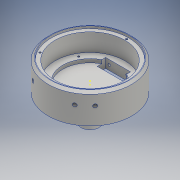
# Autodesk Inventor part: joint_read_side
Saved by Autodesk Inventor 2017 (Build 210142000, 142)
## iProperties
Created: 2017-09-26
Part Number: joint_read_side
Material: Aluminum 6061
Document SubType Name: Modeling
Designer: Thoma
Density: 2.7 g/cm^3
Appearance: Aluminum - Flat
Author: Thoma
Autodesk Inventor part; units mm, degrees
sketch "Sketch1" plane through (0, 0, 0) normal (0, 0, 1) x (1, 0, 0)
  circle A0 centre (0, 0) radius 35
  dimension "d0" = 70
  constraints: 1 centre point, 1 coincident
  measures "d0" diameter of A0
extrude "Extrusion1" add sketch "Sketch1" along normal blind 25
sketch "Sketch2" plane through (0, 0, 25) normal (0, 0, 1) x (1, 0, 0)
  circle A0 centre (0, 0) radius 23.5 construction
  line L0 (0, 0) -> (0, 47.2726) construction
  circle A1 centre (0, 0) radius 29.25
  point P0 (0, 23.5)
  dimension "d3" = 47
  dimension "d173" = 58.5
  constraints: 2 end point, 1 centre point, 1 coincident, 1 vertical, 1 vertical alignment, 2 other
  measures "d173" diameter of A1
extrude "Extrusion2" cut sketch "Sketch2" against normal blind 17
sketch "Sketch4" plane through (0, 0, 8) normal (0, 0, 1) x (1, 0, 0)
  circle A0 centre (0, 0) radius 22.8812
  point P0 (-4.25, 23.5)
  point P1 (4.25, 23.5)
  dimension "d148" = 45.7624
  constraints: 1 centre point
  measures "d148" diameter of A0
extrude "Extrusion4" cut sketch "Sketch4" against normal blind 3
ref_plane "Work Plane1" through (0, 35, 0) normal (0, 1, 0) x (-1, 0, 0)
sketch "Sketch8" plane through (0, 0, 25) normal (0, 0, 1) x (1, 0, 0)
  circle A0 centre (0, 0) radius 32.5
  dimension "d36" = 65
  constraints: 1 centre point, 1 coincident
  measures "d36" diameter of A0
extrude "Extrusion7" cut sketch "Sketch8" against normal blind 2
chamfer "Chamfer1" distance 2 angle 45 1 edges at (-35, 0, 25)
sketch "Sketch10" plane through (0, 0, 8) normal (0, 0, 1) x (1, 0, 0)
  circle A0 centre (0, 0) radius 25.881 construction
  circle A1 centre (0, 0) radius 22.8812 projected
  point P0 (0, -25.881)
  point P1 (-22.4136, 12.9405)
  point P2 (22.4136, 12.9405)
  dimension "d49" = 51.762
  dimension "d52" = 360
  constraints: 2 coincident, 1 vertical alignment, 7 other
hole "Hole3" at (0, -25.881, 8) at (-22.4136, 12.9405, 8) at (22.4136, 12.9405, 8) direction (0, 0, -1) diameter 1.6 depth 5 tip angle 118
sketch "Sketch11" plane through (0, 0, 23) normal (0, 0, 1) x (1, 0, 0)
  circle A0 centre (0, 0) radius 30.6575 construction
  point P0 (0, 30.6575)
  point P1 (-26.5502, -15.3287)
  point P2 (26.5502, -15.3288)
  dimension "d61" = 61.315
  dimension "d64" = 360
  constraints: 1 coincident, 1 vertical alignment, 6 other
hole "Hole4" at (0, 30.6575, 23) at (-26.5502, -15.3287, 23) at (26.5502, -15.3288, 23) direction (0, 0, -1) diameter 1.6 depth 5 tip angle 118
thread "Thread1" size "M1.6x0.35" class "6H" standard "ANSI Metric M Profile" full length
thread "Thread2" size "M1.6x0.35" class "6H" standard "ANSI Metric M Profile" full length
thread "Thread3" size "M1.6x0.35" class "6H" standard "ANSI Metric M Profile" full length
thread "Thread4" size "M1.6x0.35" class "6H" standard "ANSI Metric M Profile" full length
thread "Thread5" size "M1.6x0.35" class "6H" standard "ANSI Metric M Profile" full length
thread "Thread6" size "M1.6x0.35" class "6H" standard "ANSI Metric M Profile" full length
sketch "Sketch12" plane through (0, 0, 0) normal (0, 0, -1) x (-1, 0, 0)
  line L0 (0, 0) -> (0, -34.888) construction
  line L1 (0, 0) -> (-35, 0) construction
  circle A0 centre (0, 0) radius 35 construction
  line L2 (0, 0) -> (26.8116, -22.4976) construction
  line L3 (0, 0) -> (35, 0) construction
  line L4 (0, 0) -> (17.5, -30.3109) construction
  line L5 (0, 0) -> (35, 0) construction
  line L6 (0, 0) -> (-26.8116, -22.4976) construction
  line L7 (0, 0) -> (-17.5, -30.3109) construction
  dimension "d85" = 40
  dimension "d86" = 60
  constraints: 16 end point, 3 horizontal, 3 point on circle, 2 equal length, 2 symmetric about line, 1 vertical
  measures "d85" angle of L2 L3
  measures "d86" angle of L4 L5
ref_plane "Work Plane2" through (26.8116, -22.4976, 0) normal (0.7660444, -0.6427876, 0) x (0.6427876, 0.7660444, 0)
ref_plane "Work Plane3" through (17.5, -30.3109, 0) normal (0.5, -0.8660254, 0) x (0.8660254, 0.5, 0)
ref_plane "Work Plane4" through (-17.5, -30.3109, 0) normal (-0.5, -0.8660254, 0) x (0.8660254, -0.5, 0)
ref_plane "Work Plane5" through (-26.8116, -22.4976, 0) normal (-0.7660444, -0.6427876, 0) x (0.6427876, -0.7660444, 0)
sketch "Sketch13" plane through (-26.8116, -22.4976, 0) normal (-0.7660444, -0.6427876, 0) x (0.6427876, -0.7660444, 0)
  point P0 (0, 0)
  point P1 (0, 14.5)
  dimension "d87" = 14.5
  measures "d87" distance of point (0, 14.5) point (0, 0)
hole "Hole5" at (-26.8116, -22.4976, 14.5) direction (0.7660444, 0.6427876, 0) diameter 3 depth 4 tip angle 118
sketch "Sketch14" plane through (-17.5, -30.3109, 0) normal (-0.5, -0.8660254, 0) x (0.8660254, -0.5, 0)
  point P0 (0, 0)
  point P1 (0, 14.5)
  dimension "d95" = 14.5
  measures "d95" distance of point (0, 0) point (0, 14.5)
hole "Hole6" at (-17.5, -30.3109, 14.5) direction (0.5, 0.8660254, 0) diameter 3 depth 4 tip angle 118
sketch "Sketch15" plane through (17.5, -30.3109, 0) normal (0.5, -0.8660254, 0) x (0.8660254, 0.5, 0)
  point P0 (0, 0)
  point P1 (0, 14.5)
  dimension "d128" = 14.5
  measures "d128" distance of point (0, 0) point (0, 14.5)
hole "Hole9" at (17.5, -30.3109, 14.5) direction (-0.5, 0.8660254, 0) diameter 3 depth 4 tip angle 118
sketch "Sketch16" plane through (26.8116, -22.4976, 0) normal (0.7660444, -0.6427876, 0) x (0.6427876, 0.7660444, 0)
  line L0 (-4, 5) -> (4, 5) projected
  point P0 (0, 0)
  point P1 (0, 14.5)
  dimension "d129" = 14.5
  measures "d129" distance of point (0, 14.5) point (0, 0)
hole "Hole10" at (26.8116, -22.4976, 14.5) direction (-0.7660444, 0.6427876, 0) diameter 3 depth 4 tip angle 118
thread "Thread7" size "M3x0.5" class "6H" standard "ANSI Metric M Profile" full length
thread "Thread8" size "M3x0.5" class "6H" standard "ANSI Metric M Profile" full length
sketch "Sketch17" plane through (0, 0, 0) normal (0, 0, -1) x (-1, 0, 0)
  circle A0 centre (0, 0) radius 7.5
  dimension "d125" = 15
  constraints: 1 centre point, 1 coincident
  measures "d125" diameter of A0
extrude "Extrusion8" add sketch "Sketch17" along normal blind 22.2
thread "Thread11" size "M3x0.5" class "6H" standard "ANSI Metric M Profile" full length
thread "Thread12" size "M3x0.5" class "6H" standard "ANSI Metric M Profile" full length
ref_plane "Work Plane6" through (0, 35, 0) normal (0, 1, 0) x (-1, 0, 0)
sketch "Sketch21" plane through (0, 0, 8) normal (0, 0, 1) x (1, 0, 0)
  point P0 (0, 0)
sketch "Sketch22" plane through (0, 0, 5) normal (0, 0, 1) x (1, 0, 0)
  point P0 (0, 0)
sketch "Sketch23" plane through (0, 0, 8) normal (0, 0, 1) x (1, 0, 0)
  circle A0 centre (0, 0) radius 23.6
  line L0 (-10.5, 16.6) -> (10.5, 16.6)
  line L1 (10.5, 16.6) -> (10.5, 23.6)
  line L2 (10.5, 23.6) -> (-10.5, 23.6)
  line L3 (-10.5, 23.6) -> (-10.5, 16.6)
  line L4 (-10.5, 16.6) -> (10.5, 23.6) construction
  line L5 (10.5, 16.6) -> (-10.5, 23.6) construction
  point P0 (0, 20.1)
  point P1 (0, 23.6)
  dimension "d175" = 47.2
  dimension "d176" = 21
  dimension "d177" = 7
  constraints: 12 end point, 3 midpoint, 2 parallel, 1 coincident, 1 horizontal, 1 perpendicular, 1 vertical alignment, 2 other
  measures "d176" distance of L2.end L1.end
  measures "d177" distance of L1.end L0.end
extrude "Extrusion10" cut sketch "Sketch23" against normal through all contours L1 L0 L3 A0 | A0 L2 L1 | L3 L2 A0 picked at (0, 18.9333)
sketch "Sketch24" plane through (-10.5, 23.6, 8) normal (0, -1, 0) x (1, 0, 0)
  line L0 (10.5, -8) -> (10.5, 7) construction
  circle A0 centre (3, -3.9) radius 1.05 construction
  circle A1 centre (18, -3.9) radius 1.05 construction
  line L1 (-24.5, -8) -> (45.5, -8) construction
  dimension "d180" = 15
  dimension "d181" = 2.1
  dimension "d182" = 2.1
  dimension "d183" = 4.1
  dimension "d184" = 4.1
  dimension "d185" = 7.5
  dimension "d186" = 7.5
  constraints: 2 centre point, 2 end point, 1 vertical
  measures "d180" distance of L0.start L0.end
  measures "d181" diameter of A0
  measures "d182" diameter of A1
  measures "d183" distance from line of L1 A1.centre
  measures "d184" distance from line of L1 A0.centre
  measures "d185" distance from line of A1.centre L0
  measures "d186" distance from line of L0 A0.centre
hole "Hole12" at (-7.5, 23.6, 4.1) at (7.5, 23.6, 4.1) direction (0, 1, 0) diameter 2.1 end through all
ref_plane "Work Plane7" through (0, 35, 0) normal (0, 1, 0) x (-1, 0, 0)
sketch "Sketch25" plane through (0, 35, 0) normal (0, 1, 0) x (-1, 0, 0)
  spline S0 degree 7 poles (7.5, 3.05) (7.6024, 3.05) (7.7041, 3.0616) (7.8033, 3.0847) (7.8982, 3.1183) (7.9874, 3.1616) (8.0695, 3.2129) (8.2018, 3.3155) (8.2554, 3.3647) (8.3042, 3.4174) (8.3481, 3.4731) (8.3871, 3.5312) (8.421, 3.5913) (8.523, 3.8079) (8.5648, 3.9733) (8.5756, 4.1431) (8.5556, 4.3127) (8.5047, 4.4773) (8.4227, 4.6319) (8.2314, 4.8631) (8.138, 4.9501) (8.0297, 5.0258) (7.9083, 5.0862) (7.7771, 5.1283) (7.6396, 5.15) (7.3498, 5.15) (7.2021, 5.1249) (7.0619, 5.0763) (6.9338, 5.0068) (6.8212, 4.9204) (6.7266, 4.8219) (6.5522, 4.5818) (6.4825, 4.433) (6.4407, 4.2763) (6.4264, 4.1159) (6.4398, 3.9557) (6.4809, 3.7997) (6.5915, 3.5645) (6.6435, 3.479) (6.7059, 3.3979) (6.7785, 3.3228) (6.861, 3.2553) (6.9528, 3.197) (7.1111, 3.1226) (7.172, 3.099) (7.2352, 3.0796) (7.3002, 3.0649) (7.3664, 3.055) (7.4332, 3.05) (7.5, 3.05) knots 0 0 0 0 0 0 0 0 0.097814 0.097814 0.097814 0.097814 0.097814 0.097814 0.174705 0.174705 0.174705 0.174705 0.174705 0.174705 0.367929 0.367929 0.367929 0.367929 0.367929 0.367929 0.499929 0.499929 0.499929 0.499929 0.499929 0.499929 0.641888 0.641888 0.641888 0.641888 0.641888 0.641888 0.825317 0.825317 0.825317 0.825317 0.825317 0.825317 0.935792 0.935792 0.935792 0.935792 0.935792 0.935792 1 1 1 1 1 1 1 1 projected
  spline S1 degree 8 poles (-7.5, 3.05) (-7.4062, 3.05) (-7.3129, 3.0596) (-7.2213, 3.0786) (-7.1328, 3.1065) (-7.0485, 3.1428) (-6.9695, 3.1865) (-6.8967, 3.2363) (-6.7353, 3.3699) (-6.6535, 3.4592) (-6.5853, 3.5566) (-6.531, 3.6599) (-6.4904, 3.7674) (-6.4634, 3.8775) (-6.45, 3.9888) (-6.45, 4.2111) (-6.4634, 4.3224) (-6.4904, 4.4326) (-6.531, 4.5401) (-6.5853, 4.6434) (-6.6535, 4.7408) (-6.7353, 4.8302) (-6.9198, 4.9827) (-7.0217, 5.0482) (-7.135, 5.1014) (-7.2569, 5.1395) (-7.3841, 5.1603) (-7.513, 5.1631) (-7.6398, 5.1482) (-7.9497, 5.0686) (-8.1185, 4.9827) (-8.2621, 4.8681) (-8.3781, 4.7323) (-8.4648, 4.5818) (-8.522, 4.4227) (-8.55, 4.2604) (-8.55, 3.9849) (-8.5356, 3.8697) (-8.5067, 3.7558) (-8.4632, 3.6449) (-8.4051, 3.5388) (-8.3322, 3.4394) (-8.2449, 3.349) (-8.0787, 3.22) (-8.0079, 3.1744) (-7.9317, 3.1345) (-7.8507, 3.1015) (-7.7661, 3.076) (-7.6786, 3.0587) (-7.5896, 3.05) (-7.5, 3.05) knots 0 0 0 0 0 0 0 0 0 0.102088 0.102088 0.102088 0.102088 0.102088 0.102088 0.102088 0.2495 0.2495 0.2495 0.2495 0.2495 0.2495 0.2495 0.396882 0.396882 0.396882 0.396882 0.396882 0.396882 0.396882 0.534522 0.534522 0.534522 0.534522 0.534522 0.534522 0.534522 0.748413 0.748413 0.748413 0.748413 0.748413 0.748413 0.748413 0.901864 0.901864 0.901864 0.901864 0.901864 0.901864 0.901864 1 1 1 1 1 1 1 1 1 projected
  line L0 (-35, 0) -> (35, 0) projected
  line L1 (35, 23) -> (-35, 23) projected
  circle A0 centre (7.5, 4.1) radius 1.05 projected
  circle A1 centre (-7.5, 4.1) radius 1.05 projected
  line L2 (7.5, 4.1) -> (-7.5, 4.1) construction
  line L3 (7.5, 6.6) -> (-7.5, 6.6)
  line L4 (-7.5, 1.6) -> (7.5, 1.6)
  arc A2 (7.5, 1.6) -> (7.5, 6.6) centre (7.5, 4.1) ccw
  arc A3 (-7.5, 6.6) -> (-7.5, 1.6) centre (-7.5, 4.1) ccw
  point P0 (0, 0)
  point P1 (0, 4.1)
  dimension "d195" = 5
  constraints: 8 end point, 8 vertical alignment, 4 point on circle, 4 tangent, 2 centre point, 2 horizontal alignment, 1 horizontal, 1 midpoint, 1 parallel, 2 other
  measures "d195" diameter of A3
extrude "Extrusion11" cut sketch "Sketch25" against normal blind 2
body "Solid1"
